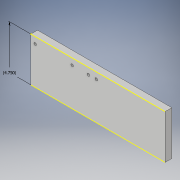
# Autodesk Inventor part: kermit bumper (Medium 4)
Saved by Autodesk Inventor 2018.2 (Build 222227000, 227)
## iProperties
Created: 2018-02-15
Part Number: kermit bumper (Medium 4)
Material: Generic
Document SubType Name: Modeling
Designer: kalra.rohan
Density: 1 g/cm^3
Appearance: Default
Author: kalra.rohan
Autodesk Inventor part; units mm, degrees
ref_plane "YZ Plane" through (0, 0, 0) normal (1, 0, 0) x (0, 1, 0)
ref_plane "XZ Plane" through (0, 0, 0) normal (0, 1, 0) x (-1, 0, 0)
ref_plane "XY Plane" through (0, 0, 0) normal (0, 0, 1) x (1, 0, 0)
sketch "Sketch1" plane through (0, 0, 0) normal (0, 0, 1) x (1, 0, 0)
  point P0 (0, 0)
sketch "Sketch2" plane through (0, 0, 0) normal (0, 0, 1) x (1, 0, 0)
  line L0 (0, 0) -> (368.3, 0)
  line L1 (368.3, 0) -> (368.3, -120.65)
  line L2 (368.3, -120.65) -> (0, -120.65)
  line L3 (0, -120.65) -> (0, 0)
  circle A0 centre (11.938, -17.78) radius 3.556
  circle A1 centre (113.284, -17.78) radius 3.556
  circle A2 centre (157.988, -17.78) radius 3.556
  circle A3 centre (179.578, -17.78) radius 3.556
  dimension "d1" = 368.3
  dimension "d2" = 120.65
  dimension "d3" = 7.112
  dimension "d4" = 11.938
  dimension "d5" = 102.87
  dimension "d6" = 7.112
  dimension "d8" = 101.346
  dimension "d9" = 7.112
  dimension "d10" = 102.87
  dimension "d11" = 44.704
  dimension "d12" = 7.112
  dimension "d13" = 102.87
  dimension "d14" = 21.59
  constraints: 8 end point, 4 centre point, 2 parallel, 1 horizontal, 1 perpendicular
  measures "d1" distance between parallel lines of L1 L3
  measures "d2" distance between parallel lines of L0 L2
  measures "d3" diameter of A0
  measures "d4" distance from line of A0.centre L3
  measures "d5" distance from line of A0.centre L2
  measures "d6" diameter of A1
  measures "d8" distance of A1.centre A0.centre
  measures "d9" diameter of A2
  measures "d10" distance from line of A2.centre L2
  measures "d11" distance of A2.centre A1.centre
  measures "d12" diameter of A3
  measures "d13" distance from line of A3.centre L2
  measures "d14" distance of A3.centre A2.centre
extrude "Extrusion1" add sketch "Sketch2" against normal blind 18.3261
sketch "Sketch3" plane through (0, 0, 0) normal (0, 0, 1) x (1, 0, 0)
  line L0 (368.3, -120.65) -> (0, -120.65) projected
  line L1 (0, 0) -> (368.3, 0) projected
  dimension "d17" = 120.65
  measures "d17" distance between parallel lines of L0 L1
body "Solid1"
